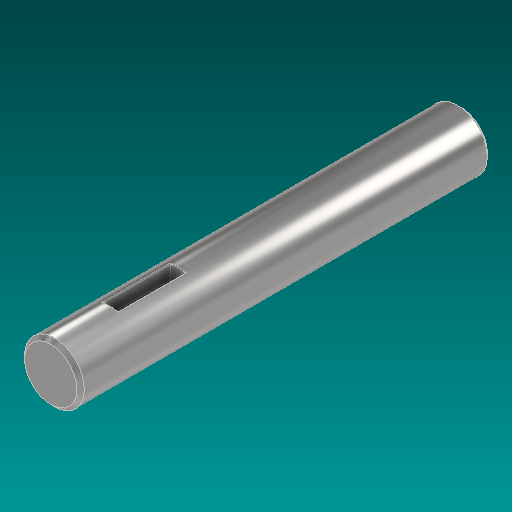
# Autodesk Inventor part: asGearbox
Saved by Autodesk Inventor 2020.3 (Build 243373000, 373)
## iProperties
Created: 2020-05-14
Part Number: asGearbox
Material: Stainless Steel
Document SubType Name: Modeling
Designer: Svend
Density: 8 g/cm^3
Appearance: Semi-Polished
Author: Svend
Autodesk Inventor part; units mm, degrees
ref_plane "YZ Plane" through (0, 0, 0) normal (1, 0, 0) x (0, 1, 0)
ref_plane "XY Plane" through (0, 0, 0) normal (0, 0, 1) x (1, 0, 0)
sketch "Sketch1" plane through (0, 0, 0) normal (0, 0, 1) x (1, 0, 0)
  circle A0 centre (0, 0) radius 4
  dimension "d0" = 8
  constraints: 1 centre point, 1 coincident
  measures "d0" diameter of A0
extrude "Extrusion1" add sketch "Sketch1" along normal mid plane 55
chamfer "Chamfer1" distance 0.5 angle 45 2 edges at (-4, 0, 27.5) (-4, 0, -27.5)
ref_plane "Work Plane1" through (0, 4, 0) normal (0, 1, 0) x (-1, 0, 0)
sketch "Sketch2" plane through (0, 4, 0) normal (0, 1, 0) x (-1, 0, 0)
  line L0 (-3.5, 27.5) -> (3.5, 27.5) projected
  line L1 (4, -27) -> (4, 27) projected
  line L2 (1, 19.5) -> (-1, 19.5)
  line L3 (-1, 19.5) -> (-1, 10.5)
  line L4 (-1, 10.5) -> (1, 10.5)
  line L5 (1, 10.5) -> (1, 19.5)
  point P0 (0, 0)
  dimension "d7" = 2
  dimension "d8" = 9
  dimension "d9" = 8
  dimension "d10" = 1
  constraints: 8 end point, 2 parallel, 1 horizontal, 1 perpendicular
  measures "d7" distance of L4.end L3.end
  measures "d8" distance of L3.end L2.end
  measures "d9" distance between parallel lines of L0 L2
  measures "d10" distance from line of point (0, 0) L5
extrude "Extrusion2" cut sketch "Sketch2" against normal blind 2
fillet "Fillet1" radius 0.1 4 edges at (1, 3.873, 15) (0, 4, 10.5) (-1, 3.873, 15) (0, 4, 19.5)
body "Solid1"
